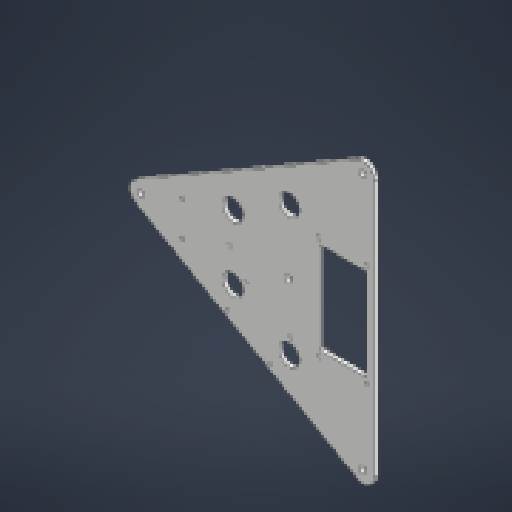
# Autodesk Inventor part: second_etage
Saved by Autodesk Inventor 2024 (Build 280153000, 153)
## iProperties
Created: 2026-03-25
Part Number: second_etage
Material: PET Plastic
Document SubType Name: Modeling
Designer: schar
Density: 1.541 g/cm^3
Appearance: Polycarbonate - Clear
Mass: 79.3801 g
Surface Area: 379.989 cm^2
Volume: 51.5121 cm^3
Author: schar
Autodesk Inventor part; units mm, degrees
ref_plane "YZ Plane" through (0, 0, 0) normal (1, 0, 0) x (0, 1, 0)
ref_plane "XZ Plane" through (0, 0, 0) normal (0, 1, 0) x (-1, 0, 0)
ref_plane "XY Plane" through (0, 0, 0) normal (0, 0, 1) x (1, 0, 0)
sketch "Sketch1" plane through (0, 0, 0) normal (0, 0, 1) x (1, 0, 0)
  line L0 (-169.4076, 105.3841) -> (50.098, -274.8108)
  circle A0 centre (-54.282, -94.0192) radius 2.75 projected
  circle A1 centre (0, 0) radius 8.5
  circle A2 centre (-162.8461, -94.0192) radius 8.5
  circle A3 centre (0, -188.0385) radius 8.5
  line L1 (0, 0) -> (0, -188.0385)
  line L2 (0, -188.0385) -> (-162.8461, -94.0192)
  line L3 (-162.8461, -94.0192) -> (0, 0)
  line L4 (38.7758, 32.2022) -> (-208.87, -110.7762)
  line L5 (8.5, -269.7975) -> (8.5, 26.6982)
  line L6 (49.2969, -226.315) -> (-222.0406, -69.6582)
  circle A4 centre (-54.282, -94.0192) radius 2.75
  point P0 (8.5, -188.0385)
  point P1 (8.5, 0)
  point P2 (-4.25, 7.3612)
  point P3 (-167.0961, -86.658)
  point P4 (-167.0961, -101.3805)
  point P5 (-4.25, -195.3997)
  dimension "d0" = 17
  dimension "d3" = 360
  dimension "d49" = 5.5
  constraints: 14 end point, 6 tangent, 4 centre point, 4 coincident, 17 other
  measures "d0" diameter of A1
  measures "d49" diameter of A4
extrude "Extrusion1" add sketch "Sketch1" along normal blind 3 contours L4 A1 L3 L0 | L0 L3 A2 L4 | L3 A1 L1 A3 L0 A0 | L0 A0 A3 L2 A2 L3 | A1 L1 L3 | A2 L3 L2 | A2 L2 L3 | L3 L1 A1 | L5 A3 L1 A1 | A2 L2 A3 L6 | A3 L0 L1 | A3 L2 L0 | A3 L1 L0 | L0 L2 A3
sketch "Sketch2" plane through (0, 0, 3) normal (0, 0, 1) x (1, 0, 0)
  circle A0 centre (0, 0) radius 2.5
  line L0 (-169.4076, 105.3841) -> (50.098, -274.8108)
  line L1 (-169.4076, -293.4225) -> (50.098, 86.7723)
  circle A1 centre (-54.282, -94.0192) radius 2.75 projected
  circle A2 centre (-162.8461, -94.0192) radius 2.5
  circle A3 centre (0, -188.0385) radius 2.5
  point P0 (-54.282, -94.0192)
  dimension "d7" = 5
  dimension "d10" = 360
  constraints: 4 end point, 3 centre point, 2 coincident, 13 other
  measures "d7" diameter of A0
extrude "Extrusion2" cut sketch "Sketch2" against normal up to surface (3 mm away) contours A0 L1 | A3 L0 | L0 A3 | L1 A0 | A2
sketch "Sketch3" plane through (0, 0, 0) normal (0, 0, -1) x (-1, 0, 0)
  circle A0 centre (54.282, -94.0192) radius 2.75 projected
  circle A1 centre (0, 0) radius 2.5 projected
  line L0 (0, 0) -> (54.282, -94.0192)
  circle A2 centre (162.8461, -94.0192) radius 2.5 projected
  line L1 (54.282, -94.0192) -> (162.8461, -94.0192)
  circle A3 centre (0, -188.0385) radius 2.5 projected
  line L2 (54.282, -94.0192) -> (0, -188.0385)
  line L3 (0, 0) -> (32.5, -56.2917)
  circle A4 centre (32.5, -56.2917) radius 1.5
  circle A5 centre (32.5, -56.2917) radius 2.5
  circle A6 centre (32.5, -131.7468) radius 2.5
  circle A7 centre (32.5, -131.7468) radius 1.5
  circle A8 centre (97.8461, -94.0192) radius 2.5
  circle A9 centre (97.8461, -94.0192) radius 1.5
  dimension "d14" = 65
  dimension "d15" = 3
  dimension "d16" = 5
  dimension "d19" = 360
  constraints: 8 end point, 6 centre point, 5 coincident, 1 horizontal, 1 point on line, 13 other
  measures "d14" distance of L0.start L3.end
  measures "d15" diameter of A4
  measures "d16" diameter of A5
extrude "Extrusion3" add sketch "Sketch3" along normal blind 3 contours A6 L2 A7 | L2 A7 A6 | A5 L0 A4 | L0 A4 A5 | A8 L1 A9 | L1 A9 A8
sketch "Sketch4" plane through (0, 0, 0) normal (0, 0, -1) x (-1, 0, 0)
  circle A0 centre (32.5, -56.2917) radius 1.5 projected
  circle A1 centre (32.5, -131.7468) radius 1.5 projected
  circle A2 centre (97.8461, -94.0192) radius 1.5 projected
  point P0 (0, 0)
extrude "Extrusion4" cut sketch "Sketch4" against normal blind 3
sketch "Sketch5" plane through (0, 0, 3) normal (0, 0, 1) x (1, 0, 0)
  circle A0 centre (-32.5, -56.2917) radius 1.5 projected
  circle A1 centre (-32.5, -131.7468) radius 1.5 projected
  line L0 (-32.5, -56.2917) -> (2.5, -56.2917)
  line L1 (2.5, -56.2917) -> (2.5, -131.7468)
  line L2 (2.5, -131.7468) -> (-32.5, -131.7468)
  line L3 (-32.5, -131.7468) -> (-32.5, -56.2917)
  circle A2 centre (2.5, -56.2917) radius 1.5
  circle A3 centre (2.5, -131.7468) radius 1.5
  point P0 (0, 0)
  dimension "d25" = 35
  dimension "d26" = 3
  dimension "d27" = 3
  constraints: 8 end point, 4 coincident, 2 centre point, 2 parallel, 1 horizontal, 1 perpendicular
  measures "d25" distance of L1.end L2.end
  measures "d26" diameter of A2
  measures "d27" diameter of A3
extrude "Extrusion5" cut sketch "Sketch5" against normal blind 3 contours A2 L1 L0 | L0 L1 A2 | A3 L2 L1 | L1 L2 A3
sketch "Sketch7" plane through (0, 0, 3) normal (0, 0, 1) x (1, 0, 0)
  circle A0 centre (-32.5, -56.2917) radius 1.5 projected
  circle A1 centre (2.5, -131.7468) radius 1.5 projected
  line L0 (-32.5, -56.2917) -> (2.5, -131.7468)
  circle A2 centre (2.5, -56.2917) radius 1.5 projected
  circle A3 centre (-32.5, -131.7468) radius 1.5 projected
  line L1 (2.5, -56.2917) -> (-32.5, -131.7468)
  line L2 (2.5, -60.5192) -> (-32.5, -60.5192)
  line L3 (-32.5, -60.5192) -> (-32.5, -127.5192)
  line L4 (-32.5, -127.5192) -> (2.5, -127.5192)
  line L5 (2.5, -127.5192) -> (2.5, -60.5192)
  line L6 (2.5, -60.5192) -> (-32.5, -127.5192) construction
  line L7 (-32.5, -60.5192) -> (2.5, -127.5192) construction
  point P0 (0, 0)
  point P1 (-15, -94.0192)
  dimension "d36" = 35
  dimension "d37" = 67
  constraints: 16 end point, 3 midpoint, 2 parallel, 1 horizontal, 1 perpendicular
  measures "d36" distance of L4.end L3.end
  measures "d37" distance of L3.end L2.end
extrude "Extrusion7" cut sketch "Sketch7" against normal blind 3 contours L2 L1 L0 | L0 L1 L4 L3 L2 | L1 L2 L5 L4 L0 | L0 L4 L1
sketch "Sketch8" plane through (0, 0, 3) normal (0, 0, 1) x (1, 0, 0)
  line L0 (-53.465, -129.8041) -> (-67.565, -154.226)
  line L1 (-67.565, -154.226) -> (-99.7811, -135.626)
  line L2 (-99.7811, -135.626) -> (-85.6811, -111.2041)
  line L3 (-85.6811, -111.2041) -> (-53.465, -129.8041)
  circle A0 centre (-67.565, -154.226) radius 1.25
  circle A1 centre (-53.465, -129.8041) radius 1.25
  circle A2 centre (-99.7811, -135.626) radius 1.25
  circle A3 centre (-85.6811, -111.2041) radius 1.25
  line L4 (-167.0961, -101.3805) -> (-4.25, -195.3997) projected
  line L5 (-167.0961, -101.3805) -> (-4.25, -195.3997) projected
  line L6 (-85.673, -148.3901) -> (-48.0406, -83.2087)
  circle A4 centre (-54.282, -94.0192) radius 2.75 projected
  point P0 (0, 0)
  point P1 (-69.573, -120.5041)
  dimension "d40" = 28.2
  dimension "d41" = 37.2
  dimension "d42" = 2.5
  dimension "d43" = 2.5
  dimension "d44" = 2.5
  dimension "d45" = 2.5
  dimension "d46" = 4
  constraints: 10 end point, 4 centre point, 4 coincident, 2 midpoint, 2 parallel, 2 perpendicular, 2 point on line
  measures "d40" distance of L1.end L2.end
  measures "d41" distance between parallel lines of L0 L2
  measures "d42" diameter of A0
  measures "d43" diameter of A1
  measures "d44" diameter of A2
  measures "d45" diameter of A3
  measures "d46" distance between parallel lines of L1 L4
extrude "Extrusion8" cut sketch "Sketch8" against normal blind 10 contours L3 A1 L0 | L0 A1 L3 | A0 L1 L0 | L0 L1 A0 | A3 L2 L3 | L3 L2 A3 | A2 L2 L1 | L1 L2 A2
sketch "Sketch9" plane through (0, 0, 3) normal (0, 0, 1) x (1, 0, 0)
  circle A0 centre (-54.282, -46.3878) radius 7.5 projected
  circle A1 centre (-95.532, -70.2035) radius 7.5 projected
  circle A2 centre (-54.282, -141.6506) radius 7.5 projected
  circle A3 centre (-95.532, -117.8349) radius 7.5 projected
  point P0 (0, 0)
extrude "Extrusion9" cut sketch "Sketch9" against normal up to surface (3 mm away)
sketch "Sketch10" plane through (0, 0, 3) normal (0, 0, 1) x (1, 0, 0)
  line L0 (-140.8461, -109.2592) -> (-140.8461, -78.7792)
  line L1 (-140.8461, -78.7792) -> (-123.0661, -78.7792)
  circle A0 centre (-131.9561, -81.3192) radius 1.27
  circle A1 centre (-131.9561, -106.7192) radius 1.27
  point P0 (0, 0)
  constraints: 4 end point, 2 centre point, 1 horizontal, 1 vertical, 7 other
extrude "Extrusion10" cut sketch "Sketch10" against normal blind 10
body "Solid1"
